Autodesk Fusion 360 part; units mm, degrees
(part 3 of 3)
  spline S37 degree 5 poles (-18.1669, 12.4082) (-18.1626, 12.3987) (-18.1539, 12.3796) (-18.1409, 12.351) (-18.1234, 12.3131) (-18.1013, 12.2658) (-18.0791, 12.2187) (-18.0567, 12.1717) (-18.034, 12.1249) (-18.0112, 12.0783) (-17.9882, 12.0319) (-17.965, 11.9857) (-17.9416, 11.9396) (-17.9181, 11.8937) (-17.8943, 11.848) (-17.8703, 11.8025) (-17.8462, 11.7572) (-17.8218, 11.712) (-17.7973, 11.667) (-17.7725, 11.6223) (-17.7476, 11.5777) (-17.7225, 11.5333) (-17.6972, 11.4892) (-17.6716, 11.4452) (-17.6459, 11.4014) (-17.62, 11.3578) (-17.5939, 11.3145) (-17.5676, 11.2713) (-17.5411, 11.2284) (-17.5144, 11.1857) (-17.4875, 11.1431) (-17.4604, 11.1008) (-17.433, 11.0588) (-17.4055, 11.0169) (-17.3778, 10.9753) (-17.3499, 10.9339) (-17.3217, 10.8928) (-17.2934, 10.8519) (-17.2648, 10.8112) (-17.2361, 10.7708) (-17.2071, 10.7306) (-17.1779, 10.6906) (-17.1485, 10.651) (-17.1188, 10.6116) (-17.089, 10.5724) (-17.0589, 10.5336) (-17.0286, 10.495) (-16.9981, 10.4566) (-16.9673, 10.4186) (-16.9364, 10.3808) (-16.9052, 10.3433) (-16.8737, 10.3062) (-16.842, 10.2694) (-16.81, 10.2329) (-16.7778, 10.1967) (-16.7453, 10.1609) (-16.7126, 10.1254) (-16.6797, 10.0902) (-16.6465, 10.0552) (-16.6131, 10.0207) (-16.5793, 9.9866) (-16.5452, 9.953) (-16.5107, 9.92) (-16.4758, 9.8875) (-16.4406, 9.8555) (-16.4051, 9.8239) (-16.3694, 9.7925) (-16.3336, 9.7615) (-16.2974, 9.7308) (-16.2609, 9.7009) (-16.2235, 9.6721) (-16.1928, 9.6504) (-16.1691, 9.6349) (-16.1531, 9.6251) (-16.145, 9.6202) knots -1 -1 -1 -1 -1 -1 -0.98571429 -0.97142857 -0.95714286 -0.94285714 -0.92857143 -0.91428571 -0.9 -0.88571429 -0.87142857 -0.85714286 -0.84285714 -0.82857143 -0.81428571 -0.8 -0.78571429 -0.77142857 -0.75714286 -0.74285714 -0.72857143 -0.71428571 -0.7 -0.68571429 -0.67142857 -0.65714286 -0.64285714 -0.62857143 -0.61428571 -0.6 -0.58571429 -0.57142857 -0.55714286 -0.54285714 -0.52857143 -0.51428571 -0.5 -0.48571429 -0.47142857 -0.45714286 -0.44285714 -0.42857143 -0.41428571 -0.4 -0.38571429 -0.37142857 -0.35714286 -0.34285714 -0.32857143 -0.31428571 -0.3 -0.28571429 -0.27142857 -0.25714286 -0.24285714 -0.22857143 -0.21428571 -0.2 -0.18571429 -0.17142857 -0.15714286 -0.14285714 -0.12857143 -0.11428571 -0.1 -0.08571429 -0.07142857 -0.05714286 -0.04285714 -0.02857143 -0.01428571 0 0 0 0 0 0
  line L37 (-16.145, 9.6202) -> (-15.7065, 9.3586)
  arc A75 (-15.4314, 8.3574) -> (-15.7065, 9.3586) centre (-16.0909, 8.7145) ccw
  arc A76 (-15.4314, 8.3574) -> (-15.8316, 7.5719) centre (0, 0) ccw
  arc A77 (-16.8033, 7.206) -> (-15.8316, 7.5719) centre (-16.5082, 7.8955) ccw
  line L38 (-16.8033, 7.206) -> (-17.2727, 7.4069)
  spline S38 degree 5 poles (-17.2727, 7.4069) (-17.2814, 7.4106) (-17.2988, 7.4178) (-17.3252, 7.4279) (-17.3608, 7.44) (-17.4061, 7.4533) (-17.4518, 7.4653) (-17.4978, 7.4765) (-17.544, 7.4872) (-17.5904, 7.4976) (-17.6368, 7.5078) (-17.6834, 7.5175) (-17.7302, 7.5266) (-17.7772, 7.5351) (-17.8244, 7.543) (-17.8718, 7.5503) (-17.9194, 7.557) (-17.9672, 7.5633) (-18.015, 7.5692) (-18.063, 7.5748) (-18.1111, 7.58) (-18.1592, 7.5848) (-18.2076, 7.5893) (-18.256, 7.5933) (-18.3045, 7.5969) (-18.3532, 7.6001) (-18.4019, 7.603) (-18.4508, 7.6055) (-18.4998, 7.6076) (-18.5488, 7.6095) (-18.5979, 7.6109) (-18.6471, 7.6121) (-18.6964, 7.6129) (-18.7458, 7.6134) (-18.7953, 7.6135) (-18.8448, 7.6134) (-18.8944, 7.6129) (-18.9441, 7.6121) (-18.9939, 7.611) (-19.0437, 7.6095) (-19.0936, 7.6078) (-19.1436, 7.6058) (-19.1936, 7.6034) (-19.2437, 7.6008) (-19.2939, 7.5979) (-19.3441, 7.5947) (-19.3943, 7.5912) (-19.4447, 7.5874) (-19.495, 7.5833) (-19.5455, 7.5789) (-19.5959, 7.5743) (-19.6465, 7.5693) (-19.6971, 7.5641) (-19.7477, 7.5587) (-19.7983, 7.5529) (-19.8491, 7.5469) (-19.8998, 7.5406) (-19.9506, 7.534) (-20.0014, 7.5272) (-20.0523, 7.5201) (-20.1032, 7.5127) (-20.1542, 7.5051) (-20.2052, 7.4972) (-20.2562, 7.489) (-20.3072, 7.4806) (-20.3583, 7.4719) (-20.4094, 7.463) (-20.4606, 7.4538) (-20.5117, 7.4443) (-20.5629, 7.4346) (-20.6142, 7.4247) (-20.6552, 7.4165) (-20.6859, 7.4103) (-20.7064, 7.4061) (-20.7167, 7.404) knots 0 0 0 0 0 0 0.01428571 0.02857143 0.04285714 0.05714286 0.07142857 0.08571429 0.1 0.11428571 0.12857143 0.14285714 0.15714286 0.17142857 0.18571429 0.2 0.21428571 0.22857143 0.24285714 0.25714286 0.27142857 0.28571429 0.3 0.31428571 0.32857143 0.34285714 0.35714286 0.37142857 0.38571429 0.4 0.41428571 0.42857143 0.44285714 0.45714286 0.47142857 0.48571429 0.5 0.51428571 0.52857143 0.54285714 0.55714286 0.57142857 0.58571429 0.6 0.61428571 0.62857143 0.64285714 0.65714286 0.67142857 0.68571429 0.7 0.71428571 0.72857143 0.74285714 0.75714286 0.77142857 0.78571429 0.8 0.81428571 0.82857143 0.84285714 0.85714286 0.87142857 0.88571429 0.9 0.91428571 0.92857143 0.94285714 0.95714286 0.97142857 0.98571429 1 1 1 1 1 1
  arc A78 (-20.7167, 7.404) -> (-21.1121, 6.187) centre (0, 0) ccw
  spline S39 degree 5 poles (-21.1121, 6.187) (-21.105, 6.1793) (-21.0909, 6.1638) (-21.0697, 6.1407) (-21.0413, 6.11) (-21.0057, 6.0718) (-20.97, 6.0339) (-20.9342, 5.9962) (-20.8982, 5.9587) (-20.8621, 5.9214) (-20.8259, 5.8844) (-20.7895, 5.8476) (-20.753, 5.811) (-20.7164, 5.7746) (-20.6797, 5.7385) (-20.6429, 5.7026) (-20.6059, 5.6669) (-20.5688, 5.6315) (-20.5315, 5.5964) (-20.4942, 5.5614) (-20.4567, 5.5267) (-20.4191, 5.4923) (-20.3813, 5.4581) (-20.3435, 5.4242) (-20.3055, 5.3905) (-20.2674, 5.3571) (-20.2292, 5.3239) (-20.1908, 5.291) (-20.1523, 5.2583) (-20.1137, 5.2259) (-20.075, 5.1938) (-20.0361, 5.162) (-19.9972, 5.1304) (-19.9581, 5.0991) (-19.9188, 5.0681) (-19.8795, 5.0374) (-19.84, 5.0069) (-19.8004, 4.9768) (-19.7607, 4.9469) (-19.7208, 4.9174) (-19.6808, 4.8881) (-19.6407, 4.8592) (-19.6005, 4.8305) (-19.5601, 4.8022) (-19.5196, 4.7742) (-19.479, 4.7465) (-19.4383, 4.7192) (-19.3974, 4.6921) (-19.3564, 4.6654) (-19.3153, 4.6391) (-19.274, 4.6131) (-19.2326, 4.5875) (-19.1911, 4.5623) (-19.1494, 4.5375) (-19.1076, 4.5131) (-19.0656, 4.489) (-19.0235, 4.4653) (-18.9813, 4.442) (-18.939, 4.419) (-18.8966, 4.3965) (-18.8539, 4.3745) (-18.8111, 4.3531) (-18.7681, 4.3324) (-18.7248, 4.3123) (-18.6814, 4.2927) (-18.6379, 4.2736) (-18.5943, 4.2548) (-18.5506, 4.2364) (-18.5068, 4.2183) (-18.4627, 4.2012) (-18.4183, 4.1854) (-18.3824, 4.1742) (-18.3551, 4.1668) (-18.3368, 4.1624) (-18.3276, 4.1603) knots -1 -1 -1 -1 -1 -1 -0.98571429 -0.97142857 -0.95714286 -0.94285714 -0.92857143 -0.91428571 -0.9 -0.88571429 -0.87142857 -0.85714286 -0.84285714 -0.82857143 -0.81428571 -0.8 -0.78571429 -0.77142857 -0.75714286 -0.74285714 -0.72857143 -0.71428571 -0.7 -0.68571429 -0.67142857 -0.65714286 -0.64285714 -0.62857143 -0.61428571 -0.6 -0.58571429 -0.57142857 -0.55714286 -0.54285714 -0.52857143 -0.51428571 -0.5 -0.48571429 -0.47142857 -0.45714286 -0.44285714 -0.42857143 -0.41428571 -0.4 -0.38571429 -0.37142857 -0.35714286 -0.34285714 -0.32857143 -0.31428571 -0.3 -0.28571429 -0.27142857 -0.25714286 -0.24285714 -0.22857143 -0.21428571 -0.2 -0.18571429 -0.17142857 -0.15714286 -0.14285714 -0.12857143 -0.11428571 -0.1 -0.08571429 -0.07142857 -0.05714286 -0.04285714 -0.02857143 -0.01428571 0 0 0 0 0 0
  line L39 (-18.3276, 4.1603) -> (-17.8298, 4.0469)
  arc A79 (-17.2587, 3.1798) -> (-17.8298, 4.0469) centre (-17.9963, 3.3157) ccw
  circle A80 centre (0, 0) radius 2.625
  dimension "d9" = 5.25
  constraint coincident A0.centre A2.centre
  measures "d9" diameter of A80
extrude "Extrude3" cut sketch "Sketch1 (2)" against normal blind 7 contours A80 in component "Spur Gear (20 teeth)"
component "Spur Gear (20 teeth)" placed x (1, 0, 0) y (0, 1, 0) z (0, 0, 1) at (0, 0, 0)
